Camera (Autodesk Fusion 360 design; units mm, degrees)
Autodesk Fusion 360 part; units mm, degrees
sketch "Cam" plane through (0, 0, 0) normal (0, 0, 1) x (1, 0, 0)
  line L0 (-62.75, 35.75) -> (62.75, 35.75)
  line L1 (62.75, 35.75) -> (62.75, -35.75)
  line L2 (62.75, -35.75) -> (-62.75, -35.75)
  line L3 (-62.75, -35.75) -> (-62.75, 35.75)
  line L4 (62.75, -35.75) -> (70.55, -35.75)
  line L5 (70.55, -35.75) -> (70.55, 1.75)
  line L6 (70.55, 1.75) -> (73.25, 4.45)
  line L7 (73.25, 4.45) -> (73.25, 35.75)
  line L8 (73.25, 35.75) -> (62.75, 35.75)
  line L9 (-62.75, 35.75) -> (62.75, -35.75) construction
  line L10 (-62.75, -35.75) -> (62.75, 35.75) construction
  dimension "d122" = 125.5
  dimension "d123" = 71.5
  dimension "d126" = 10.5
  dimension "d127" = 7.8
  dimension "d395" = 135
  dimension "d396" = 31.3
  constraint horizontal L0
  constraint vertical L1
  constraint horizontal L2
  constraint vertical L3
  constraint perpendicular L1 L4
  constraint perpendicular L4 L5
  constraint perpendicular L4 L7
  constraint perpendicular L7 L8
  constraint coincident origin L10
  constraint coincident origin L9
  measures "d122" distance of L0.start L0.end
  measures "d123" distance of L0.start L2.end
  measures "d126" distance of L0.end L7.end
  measures "d127" distance of L1.end L4.end
  measures "d395" angle of L5 L6
  measures "d396" distance of L6.end L7.end
extrude "Extrude2" add sketch "Cam" along normal blind 50 contours L0 L1 L2 L3
chamfer "Chamfer2" distance 7 angle 45 3 edges at (-62.75, 0, 50) (0, 35.75, 50) (62.75, 0, 50)
shell "Shell1" thickness 3 removed faces 1 at (20.9167, -11.9167, 0)
extrude "Extrude3" add sketch "Cam" along normal blind 14.7 contours L1 L4 L5 L6 L7 L8
sketch "Cam hole" plane through (0, -35.75, 0) normal (0, -1, 0) x (1, 0, 0)
  line L0 (62.75, 43) -> (55.75, 50)
  line L1 (55.75, 50) -> (-55.75, 50)
  line L2 (-55.75, 50) -> (-62.75, 43)
  line L3 (-62.75, 43) -> (-62.75, 0)
  line L4 (-62.75, 0) -> (70.55, 0)
  line L5 (70.55, 0) -> (70.55, 14.7)
  line L6 (70.55, 14.7) -> (62.75, 14.7)
  line L7 (62.75, 14.7) -> (62.75, 43)
  circle A0 centre (33.25, 23.5) radius 17.5
  dimension "d137" = 35
  dimension "d154" = 23.5
  dimension "d155" = 29.5
  measures "d137" diameter of A0
  measures "d154" distance of L4 A0.centre
  measures "d155" distance of L7 A0.centre
extrude "Extrude4" cut sketch "Cam hole" against normal blind 20 contours A0
sketch "Cam Fix" plane through (0, 0, 0) normal (0, 0, -1) x (1, 0, 0)
  line L0 (-59.75, -32.75) -> (-59.75, 32.75)
  line L1 (-59.75, 32.75) -> (59.75, 32.75)
  line L2 (59.75, 32.75) -> (59.75, -32.75)
  line L3 (59.75, -32.75) -> (-59.75, -32.75)
  line L4 (70.55, 35.75) -> (-62.75, 35.75)
  line L5 (-62.75, 35.75) -> (-62.75, -35.75)
  line L6 (-62.75, -35.75) -> (73.25, -35.75)
  line L7 (73.25, -35.75) -> (73.25, -4.45)
  line L8 (73.25, -4.45) -> (70.55, -1.75)
  line L9 (70.55, -1.75) -> (70.55, 35.75)
  line L10 (-59.75, 32.75) -> (-49.75, 32.75)
  line L11 (-49.75, 32.75) -> (-49.75, 22.75)
  line L12 (-49.75, 22.75) -> (-59.75, 22.75)
  line L13 (-59.75, 22.75) -> (-59.75, 32.75)
  line L14 (-59.75, -32.75) -> (-49.75, -32.75)
  line L15 (-49.75, -32.75) -> (-49.75, -22.75)
  line L16 (-49.75, -22.75) -> (-59.75, -22.75)
  line L17 (-59.75, -22.75) -> (-59.75, -32.75)
  line L18 (-59.75, 32.75) -> (-49.75, 22.75) construction
  line L19 (-59.75, -22.75) -> (-49.75, -32.75) construction
  circle A0 centre (-54.75, 27.75) radius 2.6
  circle A1 centre (64.75, 27.75) radius 2.6
  circle A2 centre (64.75, -27.75) radius 2.6
  circle A3 centre (-54.75, -27.75) radius 2.6
  line L20 (59.75, 32.75) -> (69.75, 32.75)
  line L21 (69.75, 32.75) -> (69.75, 22.75)
  line L22 (69.75, 22.75) -> (59.75, 22.75)
  line L23 (59.75, 22.75) -> (59.75, 32.75)
  line L24 (59.75, -22.75) -> (69.75, -22.75)
  line L25 (69.75, -22.75) -> (69.75, -32.75)
  line L26 (69.75, -32.75) -> (59.75, -32.75)
  line L27 (59.75, -32.75) -> (59.75, -22.75)
  line L28 (59.75, -22.75) -> (69.75, -32.75) construction
  line L29 (59.75, 32.75) -> (69.75, 22.75) construction
  dimension "d140" = 10
  dimension "d141" = 10
  dimension "d142" = 10
  dimension "d143" = 10
  dimension "d148" = 5.2
  dimension "d149" = 5.2
  dimension "d150" = 5.2
  dimension "d151" = 5.2
  dimension "d156" = 10
  dimension "d157" = 10
  dimension "d158" = 10
  dimension "d159" = 10
  constraint horizontal L10
  constraint vertical L11
  constraint horizontal L12
  constraint vertical L13
  constraint coincident L0.end L1.start
  constraint horizontal L14
  constraint vertical L15
  constraint horizontal L16
  constraint vertical L17
  constraint coincident L0.start L3.end
  constraint coincident L1.end L2.start
  constraint midpoint L18 A0.centre
  constraint midpoint L19 A3.centre
  constraint horizontal L20
  constraint vertical L21
  constraint horizontal L22
  constraint vertical L23
  constraint horizontal L24
  constraint vertical L25
  constraint horizontal L26
  constraint vertical L27
  constraint midpoint A1.centre L29
  constraint midpoint A2.centre L28
  constraint coincident L2.end L3.start
  measures "d140" distance of L0.end L10.end
  measures "d141" distance of L0.end L12.end
  measures "d142" distance of L0.start L14.end
  measures "d143" distance of L0.start L16.end
  measures "d148" diameter of A0
  measures "d149" diameter of A1
  measures "d150" diameter of A2
  measures "d151" diameter of A3
  measures "d156" distance of L1.end L20.end
  measures "d157" distance of L1.end L22.end
  measures "d158" distance of L24.start L24.end
  measures "d159" distance of L2.end L24.start
extrude "Extrude5" add sketch "Cam Fix" against normal blind 10 contours L0 L3 L14 L15 L16 L17 | L0 L1 L10 L11 L12 L13 | A0 | A3
extrude "Extrude6" cut sketch "Cam Fix" against normal blind 3.1 contours A0 | A1 | A2 | A3
equation "Trous_Vis_diam2 = 2.2 mm"
named bodies: "Cam"
